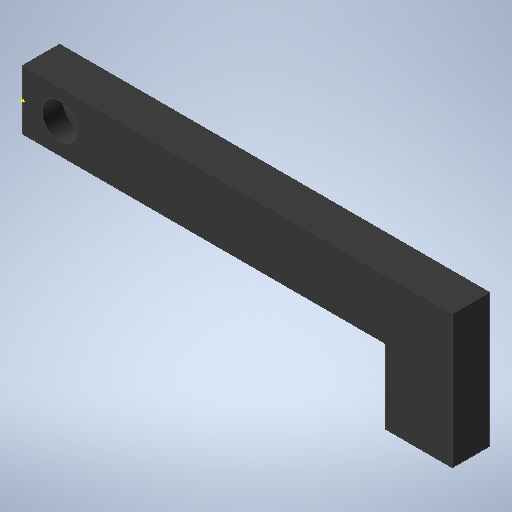
# Autodesk Inventor part: GrabberArm
Saved by Autodesk Inventor 2025.1 (Build 291241000, 241)
## iProperties
Created: 2024-11-15
Part Number: GrabberArm
Material: Generic
Document SubType Name: Modeling
Designer: 13156
Density: 1 g/cm^3
Appearance: Default
Author: 13156
Autodesk Inventor part; units mm, degrees
ref_plane "YZ Plane" through (0, 0, 0) normal (1, 0, 0) x (0, 1, 0)
ref_plane "XZ Plane" through (0, 0, 0) normal (0, 1, 0) x (-1, 0, 0)
ref_plane "XY Plane" through (0, 0, 0) normal (0, 0, 1) x (1, 0, 0)
sketch "Sketch1" plane through (0, 0, 0) normal (0, 0, 1) x (1, 0, 0)
  line L0 (0, 4) -> (55, 4)
  line L1 (55, 4) -> (55, -4)
  line L2 (55, -4) -> (0, -4)
  line L3 (0, -4) -> (0, 4)
  point P0 (0, 0)
  point P1 (27.5, -4)
  point P2 (27.5, 4)
  dimension "d0" = 55
  dimension "d1" = 8
  dimension "d4" = 4
  dimension "d5" = 0
  constraints: 8 end point, 2 midpoint, 2 parallel, 1 horizontal, 1 perpendicular
  measures "d0" distance of L0.start L0.end
  measures "d1" distance of point (27.5, -4) point (27.5, 4)
  measures "d4" distance from line of point (0, 0) L0
  measures "d5" distance from line of point (0, 0) L3
extrude "Extrusion1" add sketch "Sketch1" along normal blind 5
sketch "Sketch2" plane through (0, 0, 5) normal (0, 0, 1) x (1, 0, 0)
  point P0 (0, 0)
sketch "Sketch3" plane through (0, 0, 5) normal (0, 0, 1) x (1, 0, 0)
  circle A0 centre (5, 0) radius 2.405
  line L0 (0, 4) -> (0, -4) projected
  point P0 (0, 0)
  point P1 (0, 0)
  dimension "d6" = 4.81
  dimension "d7" = 5
  constraints: 1 centre point, 1 midpoint
  measures "d6" diameter of A0
  measures "d7" distance of point (0, 0) A0.centre
extrude "Extrusion2" cut sketch "Sketch3" against normal blind 2.8
sketch "Sketch5" plane through (0, 0, 0) normal (0, 0, -1) x (-1, 0, 0)
  line L0 (-55, 4) -> (0, 4) projected
  line L1 (-49, 4) -> (-58, 4)
  line L2 (-58, 4) -> (-58, -14)
  line L3 (-58, -14) -> (-49, -14)
  line L4 (-49, -14) -> (-49, 4)
  line L5 (-55, -4) -> (-55, 4) projected
  point P0 (0, 0)
  point P1 (-53.5, 4)
  point P2 (-53.5, -14)
  dimension "d19" = 6
  dimension "d20" = 3
  dimension "d21" = 18
  constraints: 8 end point, 2 midpoint, 2 parallel, 1 horizontal, 1 perpendicular, 1 point on line
  measures "d19" distance between parallel lines of L5 L4
  measures "d20" distance between parallel lines of L2 L5
  measures "d21" distance of point (-53.5, 4) point (-53.5, -14)
extrude "Extrusion4" add sketch "Sketch5" against normal up to surface (5 mm away)
body "Solid1"
